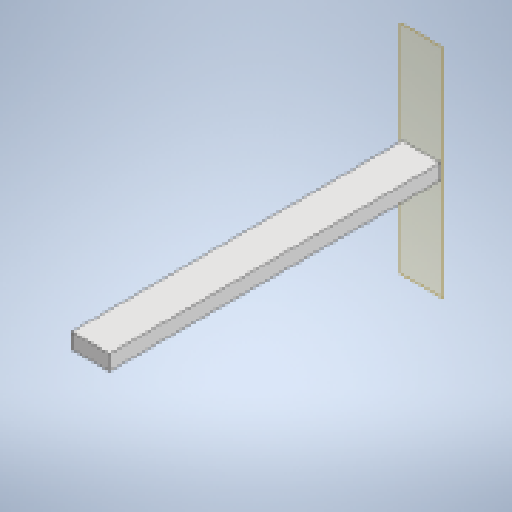
# Autodesk Inventor part: Tirante
Saved by Autodesk Inventor 2024 (Build 280153000, 153)
## iProperties
Created: 2025-03-04
Part Number: Tirante
Material: Genérico
Document SubType Name: Modeling
Designer: sergi
Density: 1 g/cm^3
Appearance: Valor por defecto
Author: sergi
Autodesk Inventor part; units mm, degrees
ref_plane "YZ Plane" through (0, 0, 0) normal (1, 0, 0) x (0, 1, 0)
ref_plane "XZ Plane" through (0, 0, 0) normal (0, 1, 0) x (-1, 0, 0)
ref_plane "Plano de trabajo1" through (0, 0, 0) normal (0, 0, 1) x (1, 0, 0)
sketch "Boceto1" plane through (0, 0, 0) normal (0, 0, 1) x (1, 0, 0)
  line L0 (10, 5) -> (0, 5) projected
  line L1 (10, 5) -> (10, 56.9) projected
  line L2 (0, 56.9) -> (10, 56.9) projected
  line L3 (0, 5) -> (0, 56.9) projected
  line L4 (10, 5) -> (0, 56.9)
  line L5 (10, 32.95) -> (0, 32.95)
  line L6 (0, 32.95) -> (0, 28.95)
  line L7 (0, 28.95) -> (10, 28.95)
  line L8 (10, 28.95) -> (10, 32.95)
  line L9 (10, 32.95) -> (0, 28.95) construction
  line L10 (0, 32.95) -> (10, 28.95) construction
  point P0 (0, 0)
  point P1 (5, 30.95)
  point P2 (0, 32.95)
  dimension "d0" = 10
  dimension "d1" = 4
  constraints: 14 end point, 3 midpoint, 2 parallel, 1 horizontal, 1 perpendicular
  measures "d0" distance of L7.end L6.end
  measures "d1" distance of L6.end L5.end
ref_plane "Plano de trabajo2" through (0, 5.3078, 87) normal (0, 0, -1) x (0, 1, 0)
extrude "Extrusión1" add sketch "Boceto1" along normal up to surface (87 mm away) contours L7 L4 L5 L1 | L7 L3 L5 L4
